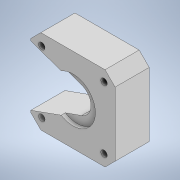
# Autodesk Inventor part: motor_spacer
Saved by Autodesk Inventor 2020.3 (Build 243373000, 373)
## iProperties
Created: 2020-11-28
Part Number: motor_spacer
Material: Generic
Document SubType Name: Modeling
Designer: Martijn
Density: 1 g/cm^3
Appearance: Default
Author: Martijn
Autodesk Inventor part; units mm, degrees
ref_plane "YZ Plane" through (0, 0, 0) normal (1, 0, 0) x (0, 1, 0)
ref_plane "XZ Plane" through (0, 0, 0) normal (0, 1, 0) x (-1, 0, 0)
ref_plane "XY Plane" through (0, 0, 0) normal (0, 0, 1) x (1, 0, 0)
sketch "Sketch1" plane through (0, 0, 0) normal (0, 0, 1) x (1, 0, 0)
  line L0 (-21, 21) -> (21, 21)
  line L1 (21, 21) -> (21, -21)
  line L2 (21, -21) -> (-21, -21)
  line L3 (-21, -21) -> (-21, -15)
  arc A0 (2.3711, -6.5862) -> (2.3711, 6.5862) centre (0, 0) ccw
  line L4 (2.3711, 6.5862) -> (-21, 15)
  line L5 (-21, 15) -> (-21, 21)
  line L6 (2.3711, -6.5862) -> (-21, -15)
  line L7 (0, -29.4) -> (0, 29.4) projected
  line L8 (-29.4, 0) -> (29.4, 0) projected
  circle A1 centre (-15.5, 15.5) radius 1.6
  circle A2 centre (15.5, 15.5) radius 1.6
  circle A3 centre (15.5, -15.5) radius 1.6
  circle A4 centre (-15.5, -15.5) radius 1.6
  dimension "d0" = 21
  dimension "d1" = 21
  dimension "d2" = 21
  dimension "d3" = 21
  dimension "d4" = 7
  dimension "d5" = 15.5
  dimension "d6" = 15.5
  dimension "d7" = 15.5
  dimension "d8" = 15.5
  dimension "d9" = 15.5
  dimension "d10" = 15.5
  dimension "d11" = 15.5
  dimension "d12" = 15.5
  dimension "d13" = 3.2
  dimension "d14" = 6
  constraints: 14 end point, 5 centre point, 3 equal radius, 3 perpendicular, 2 collinear, 2 point on circle, 2 tangent, 1 coincident, 1 horizontal, 1 vertical
  measures "d0" distance between parallel lines of L7 L5
  measures "d1" distance between parallel lines of L7 L1
  measures "d2" distance between parallel lines of L8 L0
  measures "d3" distance between parallel lines of L2 L8
  measures "d4" radius of A0
  measures "d5" distance from line of L8 A1.centre
  measures "d6" distance from line of L7 A1.centre
  measures "d7" distance from line of L8 A2.centre
  measures "d8" distance from line of L7 A2.centre
  measures "d9" distance from line of L8 A3.centre
  measures "d10" distance from line of A3.centre L7
  measures "d11" distance from line of L8 A4.centre
  measures "d12" distance from line of L7 A4.centre
  measures "d13" diameter of A1
  measures "d14" distance of L4.end L0.start
extrude "Extrusion1" add sketch "Sketch1" along normal blind 17 contours L0 L7 L4 L5 | L0 L1 L8 A0 L4 L7 | L1 L2 L7 L6 A0 L8 | L7 L2 L3 L6
chamfer "Chamfer1" distance 5 angle 45 4 edges at (-21, 21, 8.5) (-21, -21, 8.5) (21, 21, 8.5) (21, -21, 8.5)
sketch "Sketch2" plane through (0, 0, 17) normal (0, 0, 1) x (1, 0, 0)
  circle A0 centre (0, 0) radius 11.2
  dimension "d20" = 22.4
  constraints: 1 centre point, 1 coincident
  measures "d20" diameter of A0
extrude "Extrusion2" cut sketch "Sketch2" against normal blind 2
body "Solid1"
